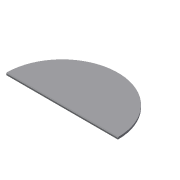
# Autodesk Inventor part: shelf-backplate
Saved by Autodesk Inventor 2022 (Build 260148000, 148)
## iProperties
Created: 2007-01-15
Part Number: shelf-backplate
Document SubType Name: Modeling
Designer: ceirmann
Density: 1 g/cm^3
Material: Generic
Appearance: Default
Author: ceirmann
Autodesk Inventor part; units mm, degrees
ref_plane "YZ Plane" through (0, 0, 0) normal (1, 0, 0) x (0, 1, 0)
ref_plane "XZ Plane" through (0, 0, 0) normal (0, 1, 0) x (-1, 0, 0)
ref_plane "XY Plane" through (0, 0, 0) normal (0, 0, 1) x (1, 0, 0)
sketch "Sketch1" plane through (0, 0, 0) normal (0, 0, 1) x (1, 0, 0)
  line L0 (0, 0) -> (203.2, 0)
  line L1 (203.2, 0) -> (203.2, 7.62)
  line L2 (203.2, 7.62) -> (0, 7.62)
  line L3 (0, 7.62) -> (0, 0)
  dimension "d0" = 7.62
  dimension "d1" = 203.2
  constraints: 8 end point, 2 parallel, 1 horizontal, 1 perpendicular
  measures "d0" distance of L2.end L0.start
  measures "d1" distance of L0.start L0.end
revolve "Revolution1" add sketch "Sketch1" angle 180 about axis through (0, 7.62, 0) along (0, 1, 0)
chamfer "Chamfer1" distance 2.54 angle 45 1 edges at (-101.6, 7.62, 0)
body "Solid1"
